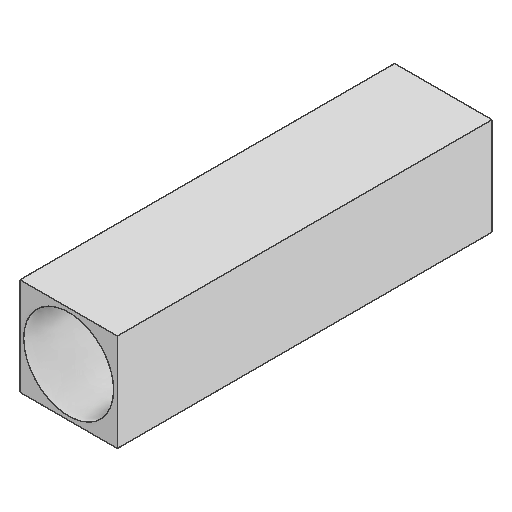
# Autodesk Inventor part: beam_pipe
Saved by Autodesk Inventor 2025.1 (Build 291241020, 241B)
## iProperties
Created: 2026-03-07
Part Number: beam_pipe
Material: Generic
Document SubType Name: Modeling
Designer: Daniel
Density: 1 g/cm^3
Appearance: Default
Author: Daniel
Autodesk Inventor part; units mm, degrees
ref_plane "YZ Plane" through (0, 0, 0) normal (1, 0, 0) x (0, 1, 0)
ref_plane "XZ Plane" through (0, 0, 0) normal (0, 1, 0) x (-1, 0, 0)
ref_plane "XY Plane" through (0, 0, 0) normal (0, 0, 1) x (1, 0, 0)
sketch "Sketch1" plane through (0, 0, 0) normal (0, 0, 1) x (1, 0, 0)
  circle A0 centre (0, 0) radius 0.06
  line L0 (-0.065, 0.065) -> (0.065, 0.065)
  line L1 (0.065, 0.065) -> (0.065, -0.065)
  line L2 (0.065, -0.065) -> (-0.065, -0.065)
  line L3 (-0.065, -0.065) -> (-0.065, 0.065)
  line L4 (-0.065, 0.065) -> (0.065, -0.065) construction
  line L5 (0.065, 0.065) -> (-0.065, -0.065) construction
  dimension "d0" = 0.12
  dimension "d2" = 0.13
  constraints: 12 end point, 2 midpoint, 2 parallel, 2 perpendicular, 1 centre point, 1 coincident, 1 horizontal
  measures "d0" diameter of A0
  measures "d2" distance of L0.start L0.end
extrude "Extrusion1" add sketch "Sketch1" along normal mid plane 0.5
body "Solid1"
